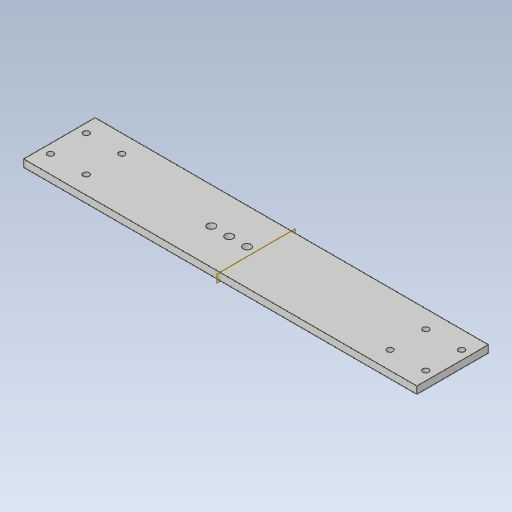
# Autodesk Inventor part: Y crossmember
Saved by Autodesk Inventor 2020 (Build 240168000, 168)
## iProperties
Created: 2019-02-27
Part Number: Y crossmember
Material: Generic
Document SubType Name: Modeling
Designer: LillaHunden
Density: 1 g/cm^3
Appearance: Default
Author: LillaHunden
Autodesk Inventor part; units mm, degrees
ref_plane "YZ Plane" through (0, 0, 0) normal (1, 0, 0) x (0, 1, 0)
ref_plane "XZ Plane" through (0, 0, 0) normal (0, 1, 0) x (-1, 0, 0)
ref_plane "XY Plane" through (0, 0, 0) normal (0, 0, 1) x (1, 0, 0)
sketch "Sketch1" plane through (0, 0, 0) normal (1, 0, 0) x (0, 1, 0)
  line L0 (2, -20) -> (-2, -20)
  line L1 (-2, -20) -> (-2, 20)
  line L2 (-2, 20) -> (2, 20)
  line L3 (2, 20) -> (2, -20)
  line L4 (2, -20) -> (-2, 20) construction
  line L5 (-2, -20) -> (2, 20) construction
  point P0 (0, 0)
  dimension "d0" = 4
  dimension "d1" = 40
  constraints: 12 end point, 2 midpoint, 2 parallel, 1 horizontal, 1 perpendicular
  measures "d0" distance of L1.end L2.end
  measures "d1" distance of L0.end L1.end
extrude "Extrusion1" add sketch "Sketch1" along normal blind 220
sketch "Sketch2" plane through (0, 2, 20) normal (0, 1, 0) x (1, 0, 0)
  point P0 (25, 30)
  point P1 (25, 10)
  point P2 (5, 10)
  point P3 (5, 30)
  point P4 (195, 30)
  point P5 (195, 10)
  point P6 (215, 10)
  point P7 (215, 30)
hole "Hole1" at (25, 2, -10) at (25, 2, 10) at (5, 2, 10) at (5, 2, -10) at (195, 2, -10) at (195, 2, 10) at (215, 2, 10) at (215, 2, -10) direction (0, -1, 0) diameter 3.4 depth 4
ref_plane "Work Plane1" through (110, 0, 0) normal (-1, 0, 0) x (0, 0, 1)
sketch "Sketch3" plane through (0, -2, -20) normal (0, -1, 0) x (1, 0, 0)
  point P0 (85, 20)
  point P1 (95, 20)
  point P2 (105, 20)
hole "Hole3" at (85, -2, 0) at (95, -2, 0) at (105, -2, 0) direction (0, 1, 0) diameter 4.5 depth 4
body "Solid1"
